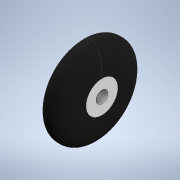
# Autodesk Inventor part: Wheel
Saved by Autodesk Inventor 2021 (Build 250183000, 183)
## iProperties
Created: 2020-11-24
Part Number: Wheel
Material: Generic
Document SubType Name: Modeling
Designer: Kanenas
Mass: 1 g
Surface Area: 9.86413 cm^2
Volume: 1.81481 cm^3
Density: 0.551021 g/cm^3
Appearance: Default
Author: Kanenas
Autodesk Inventor part; units mm, degrees
ref_plane "YZ Plane" through (0, 0, 0) normal (1, 0, 0) x (0, 1, 0)
ref_plane "XZ Plane" through (0, 0, 0) normal (0, 1, 0) x (-1, 0, 0)
ref_plane "XY Plane" through (0, 0, 0) normal (0, 0, 1) x (1, 0, 0)
sketch "Sketch1" plane through (0, 0, 0) normal (0, 0, 1) x (1, 0, 0)
  line L0 (-3, 1.5) -> (-3, 4)
  line L1 (-3, 4) -> (-3, 8) construction
  line L2 (-3, 8) -> (-1.5, 11) construction
  line L3 (-1.5, 11) -> (0, 11) construction
  spline S0 degree 3 poles (-3, 4) (-3, 8) (-1.5, 11) (0, 11) (1.5, 11) (3, 8) (3, 4) knots 1 1 1 1 2 3 4 5 5 5 5
  line L4 (-3, 1.5) -> (0, 1.5)
  line L5 (0, 11) -> (0, 1.5) construction
  line L6 (3, 1.5) -> (3, 4)
  line L7 (3, 1.5) -> (0, 1.5)
  line L8 (0, 11) -> (1.5, 11) construction
  line L9 (1.5, 11) -> (3, 8) construction
  line L10 (3, 8) -> (3, 4) construction
  line L11 (0, 1.5) -> (0, 0)
  line L12 (-2, 0) -> (2, 0)
  dimension "d0" = 3
  dimension "d1" = 2.5
  dimension "d2" = 1.5
  dimension "d4" = 3
  dimension "d5" = 4
  dimension "d6" = 1.5
  dimension "d7" = 6
  constraints: 14 end point, 4 symmetric about line, 3 horizontal, 2 vertical, 1 perpendicular, 3 other
  measures "d0" distance of L0.start L4.end
  measures "d1" distance of L0.start L0.end
  measures "d2" distance of L4.end L11.end
  measures "d4" vertical distance of L1.end L2.end
  measures "d5" distance of L0.end L1.end
  measures "d6" distance of L2.end L3.end
  measures "d7" distance of L9.end L1.end
revolve "Revolution1" add sketch "Sketch1" angle 360 about axis through (-2, 0, 0) along (1, 0, 0)
body "Solid1"
